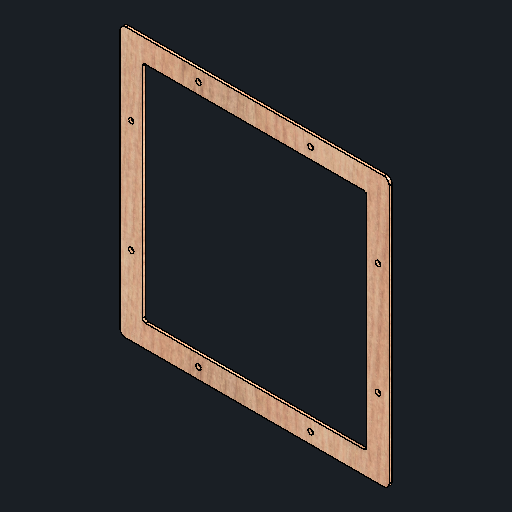
# Autodesk Inventor part: Part1
Saved by Autodesk Inventor 2026.2 (Build 302298000, 298)
## iProperties
Created: 2026-06-15
Part Number: Part1
Material: Wood (Birch)
Document SubType Name: Modeling
Designer: JoshuaEah
Density: 0.55 g/cm^3
Appearance: Birch - Natural Polished
Author: JoshuaEah
Autodesk Inventor part; units mm, degrees
ref_plane "YZ Plane" through (0, 0, 0) normal (1, 0, 0) x (0, 1, 0)
ref_plane "XZ Plane" through (0, 0, 0) normal (0, 1, 0) x (-1, 0, 0)
ref_plane "XY Plane" through (0, 0, 0) normal (0, 0, 1) x (1, 0, 0)
sketch "Sketch1" plane through (0, 0, 0) normal (0, 0, 1) x (1, 0, 0)
  line L0 (0, 0) -> (303.2125, 0)
  line L1 (303.2125, 0) -> (303.2125, 303.2125)
  line L2 (303.2125, 303.2125) -> (0, 303.2125)
  line L3 (0, 303.2125) -> (0, 0)
  line L4 (25.4, 277.8125) -> (277.8125, 277.8125)
  line L5 (277.8125, 277.8125) -> (277.8125, 25.4)
  line L6 (277.8125, 25.4) -> (25.4, 25.4)
  line L7 (25.4, 25.4) -> (25.4, 277.8125)
  line L8 (25.4, 151.6062) -> (277.8125, 151.6063)
  line L9 (151.6062, 277.8125) -> (151.6062, 25.4)
  line L10 (25.4, 277.8125) -> (277.8125, 25.4)
  point P0 (12.7, 214.7094)
  point P1 (12.7, 88.5031)
  point P2 (290.5125, 214.7094)
  point P3 (290.5125, 88.5031)
  point P4 (88.5031, 290.5125)
  point P5 (214.7094, 290.5125)
  point P6 (88.5031, 12.7)
  point P7 (214.7094, 12.7)
  dimension "d0" = 303.2125
  dimension "d19" = 25.4
  dimension "d20" = 25.4
  dimension "d21" = 25.4
  dimension "d22" = 25.4
  dimension "d25" = 12.7
  dimension "d27" = 126.2062
  constraints: 22 end point, 7 symmetric about line, 4 midpoint, 4 parallel, 3 perpendicular, 2 horizontal, 1 coincident
  measures "d0" distance of L1.end L2.end
  measures "d19" distance between parallel lines of L3 L7
  measures "d20" distance between parallel lines of L2 L4
  measures "d21" distance between parallel lines of L1 L5
  measures "d22" distance between parallel lines of L0 L6
  measures "d25" distance from line of L7 point (12.7, 214.709)
  measures "d27" diameter of point (12.7, 214.709) L8
extrude "Extrusion1" add sketch "Sketch1" against normal blind 3.175
hole "Dowel Mounting Holes" at (12.7, 214.7094, 0) at (12.7, 88.5031, 0) at (290.5125, 214.7094, 0) at (290.5125, 88.5031, 0) at (88.5031, 290.5125, 0) at (214.7094, 290.5125, 0) at (88.5031, 12.7, 0) at (214.7094, 12.7, 0) direction (0, 0, -1) diameter 6 end through all
fillet "Fillet1" radius 6.35 4 edges at (0, 303.2125, -1.5875) (303.2125, 303.2125, -1.5875) (0, 0, -1.5875) (303.2125, 0, -1.5875)
fillet "Fillet1" radius 3.175 4 edges at (277.8125, 25.4, -1.5875) (277.8125, 277.8125, -1.5875) (25.4, 277.8125, -1.5875) (25.4, 25.4, -1.5875)
equation "\"d20\" = d19"
equation "\"d21\" = d19"
equation "\"d22\" = d20"
equation "\"d25\" = 0.5 * d19"
equation "\"d27\" = -d19 + 0.5 * d0"
body "Solid1"
